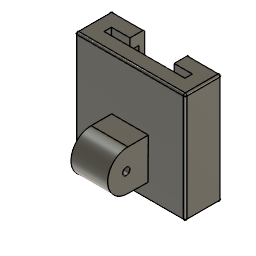
seminaire_FISA-A3_pousse-seringue (Autodesk Fusion 360 design; units mm, degrees)
part number: 2026-07-28-09-06-19-304
Autodesk Fusion 360 part; units mm, degrees
sketch "Esquisse1" plane through (0, 0, 0) normal (0, 0, 1) x (1, 0, 0)
  line L0 (20, 25) -> (50, 25)
  line L1 (50, 25) -> (50, 15)
  line L2 (50, 15) -> (20, 15)
  line L3 (20, 15) -> (20, 25)
  line L4 (24.0203, 20.9447) -> (46.0203, 20.9447)
  line L5 (46.0203, 20.9447) -> (46.0203, 18.9447)
  line L6 (46.0203, 18.9447) -> (24.0203, 18.9447)
  line L7 (24.0203, 18.9447) -> (24.0203, 20.9447)
  line L8 (29.0433, 20.9447) -> (41.0433, 20.9447)
  line L9 (41.0433, 20.9447) -> (41.0433, 25)
  line L10 (41.0433, 25) -> (29.0433, 25)
  line L11 (29.0433, 25) -> (29.0433, 20.9447)
  line L12 (30, 15) -> (40, 15)
  line L13 (40, 15) -> (40, 11)
  line L14 (40, 11) -> (30, 11)
  line L15 (30, 11) -> (30, 15)
  line L16 (36, 20.6787) -> (34, 20.6787)
  line L17 (34, 20.6787) -> (34, 25)
  line L18 (34, 25) -> (36, 25)
  line L19 (36, 25) -> (36, 20.6787)
  dimension "d1" = 10
  dimension "d2" = 30
  dimension "d3" = 22
  dimension "d4" = 2
  dimension "d5" = 4.0553
  dimension "d6" = 12
  constraint horizontal L0
  constraint vertical L1
  constraint horizontal L2
  constraint vertical L3
  constraint horizontal L4
  constraint vertical L5
  constraint horizontal L6
  constraint vertical L7
  constraint horizontal L8
  constraint vertical L9
  constraint horizontal L10
  constraint vertical L11
  constraint coincident L0 L9.end
  constraint coincident L4 L8.start
  constraint horizontal L12
  constraint vertical L13
  constraint horizontal L14
  constraint vertical L15
  constraint coincident L2 L12.start
  constraint horizontal L16
  constraint vertical L17
  constraint horizontal L18
  constraint vertical L19
  constraint coincident L0 L17.end
  measures "d1" distance of L0.end L1.end
  measures "d2" distance of L1.end L2.end
  measures "d3" distance of L5.end L6.end
  measures "d4" distance of L4.end L5.end
  measures "d5" distance of L8.end L9.end
  measures "d6" distance of L9.end L10.end
extrude "Extrusion1" add sketch "Esquisse1" along normal blind 30 contours L0 L1 L2 L3 L4 L5 L6 L7 L9 L11 L12 makes body 1
extrude "Extrusion3" add sketch "Esquisse1" along normal blind 10 contours L0 L4 L8 L10 L11 L17 | L0 L4 L8 L10 L17 L18 L19 | L0 L4 L8 L9 L10 L19 bodies 1
extrude "Extrusion4" add sketch "Esquisse1" along normal blind 2 contours L4 L5 L6 L7 L8 L16 L17 L19 | L4 L8 L16 L17 L19 bodies 1
extrude "Extrusion5" cut sketch "Esquisse1" along normal blind 11 and the other way blind -4 contours L0 L4 L8 L10 L17 L18 L19 | L4 L8 L16 L17 L19 bodies 1
fillet "Congé1" radius 0.5 10 edges at (35, 15, 30) (50, 20, 30) (50, 15, 15) (50, 25, 15) (45.5217, 25, 30) (24.5217, 25, 30) (20, 20, 30) (20, 25, 15) (35, 25, 0) (50, 20, 0) on bodies 1
fillet "Congé2" radius 0.5 6 edges at (20, 19.75, 0) (20.1464, 24.8536, 0.1464) (20, 15, 14.75) (20.1464, 15.1464, 29.8536) (49.8536, 15.1464, 0.1464) (34.75, 15, 0) on bodies 1
sketch "Esquisse3" plane through (0, 0, 0) normal (1, 0, 0) x (0, 1, 0)
  circle A0 centre (9.4258, 10.0627) radius 5.5
  line L0 (9.4258, 15.5627) -> (15, 15.5627)
  line L1 (15, 15.5627) -> (14.9253, 9.989)
  line L2 (9.4277, 4.5627) -> (14.9253, 4.4891)
  line L3 (14.9253, 4.4891) -> (14.9253, 9.989)
  dimension "d26" = 11
  constraint coincident A0 L0.start
  constraint tangent A0 L0
  constraint horizontal L0
  constraint coincident A0 L1.end
  constraint tangent A0 L1
  constraint coincident A0 L2.start
  constraint perpendicular L1 L2
  constraint vertical L3
  measures "d26" diameter of A0
extrude "Extrusion8" add sketch "Esquisse3" along normal blind 40 and the other way blind -30 separate body makes body 2
sketch "Esquisse4" plane through (0, 0, 0) normal (1, 0, 0) x (0, 1, 0)
  circle A0 centre (9, 10) radius 0.975
  dimension "d36" = 1.95
  measures "d36" diameter of A0
extrude "Extrusion9" cut sketch "Esquisse4" along normal blind 40 and the other way blind -30 bodies 2
sketch "Esquisse5" plane through (0, 0, 10) normal (0, 0, 1) x (-1, 0, 0)
  line L0 (-34, -20.9447) -> (-34, -25)
  line L1 (-34, -25) -> (-29.0433, -25)
  line L2 (-29.0433, -25) -> (-29.0433, -20.9447)
  line L3 (-29.0433, -20.9447) -> (-34, -20.9447)
  line L4 (-49, -17.8545) -> (-20, -17.8545)
  line L5 (-20, -17.8545) -> (-20, -23.3545)
  line L6 (-20, -23.3545) -> (-49, -23.3545)
  line L7 (-49, -23.3545) -> (-49, -17.8545)
  dimension "d45" = 29
  dimension "d46" = 5.5
  constraint horizontal L4
  constraint vertical L5
  constraint horizontal L6
  constraint vertical L7
  measures "d45" distance of L5.end L6.end
  measures "d46" distance of L4.end L5.end
extrude "Extrusion10" cut sketch "Esquisse5" along normal blind 17 and the other way blind -14 contours L0 L2 L3 L4 L5 L6 L7 bodies 1
